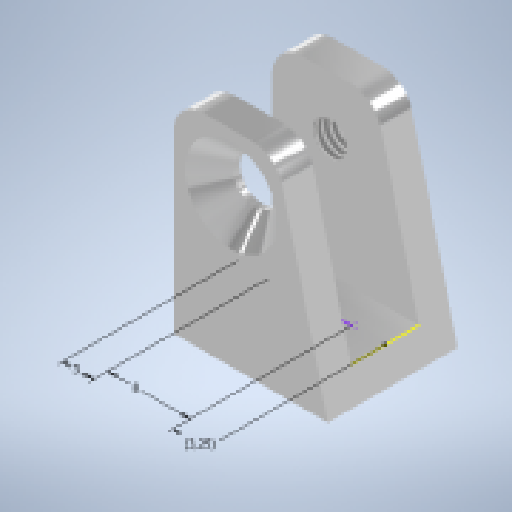
# Autodesk Inventor part: HalterUmlenkrolleH
Saved by Autodesk Inventor 2025 (Build 290162010, 162A)
## iProperties
Created: 2024-11-18
Part Number: HalterUmlenkrolleH
Material: Aluminium 6061(1)
Document SubType Name: Modeling
Designer: Admin
Density: 2.7 g/cm^3
Appearance: Aluminium - flach(1)
Author: Admin
Autodesk Inventor part; units mm, degrees
ref_plane "YZ Plane" through (0, 0, 0) normal (1, 0, 0) x (0, 1, 0)
ref_plane "XZ Plane" through (0, 0, 0) normal (0, 1, 0) x (-1, 0, 0)
ref_plane "XY Plane" through (0, 0, 0) normal (0, 0, 1) x (1, 0, 0)
sketch "Skizze1" plane through (0, 0, 0) normal (0, 0, 1) x (1, 0, 0)
  line L0 (17.8939, 18.6723) -> (2.8939, 18.6723)
  line L1 (2.8939, 18.6723) -> (2.8939, 15.6723)
  line L2 (2.8939, 15.6723) -> (17.8939, 15.6723)
  line L3 (17.8939, 15.6723) -> (17.8939, 18.6723)
  line L4 (17.8939, 9.0723) -> (2.8939, 9.0723)
  line L5 (2.8939, 9.0723) -> (2.8939, 6.0723)
  line L6 (2.8939, 6.0723) -> (17.8939, 6.0723)
  line L7 (17.8939, 6.0723) -> (17.8939, 9.0723)
  line L8 (17.8939, 15.6723) -> (17.8939, 12.3723) construction
  line L9 (17.8939, 12.3723) -> (17.8939, 9.0723) construction
  point P0 (0, 0)
  point P1 (10.3939, 9.0723)
  dimension "d0" = 15
  dimension "d1" = 3
  dimension "d2" = 3
  dimension "d3" = 6.6
  constraints: 20 end point, 5 equal length, 3 horizontal, 2 collinear, 2 perpendicular, 2 vertical, 1 midpoint
  measures "d0" distance of L2.end L1.end
  measures "d1" distance of L0.end L1.end
  measures "d2" distance of L4.end L5.end
  measures "d3" distance from line of point (10.394, 9.072) L2
extrude "Extrusion1" add sketch "Skizze1" along normal blind 20
chamfer "Fasen1" distance 5 distance2 20 1 edges at (17.8939, 7.5723, 20) measured on face at (17.3939, 7.5723, 20)
chamfer "Fasen2" distance 5 distance2 20 1 edges at (17.8939, 17.1723, 20) measured on face at (17.3939, 17.1723, 20)
fillet "Rundung1" radius 3 4 edges at (2.8939, 17.1723, 20) (2.8939, 7.5723, 20) (12.894, 17.1723, 20) (12.894, 7.5723, 20)
sketch "Skizze2" plane through (2.8939, 6.0723, 0) normal (0, -1, 0) x (1, 0, 0)
  circle A0 centre (5.6155, 14.3845) radius 5.6155 construction
  line L0 (0, 0) -> (0, 20) construction
  line L1 (5.6155, 14.3845) -> (5.6155, 20)
  line L2 (5.6155, 14.3845) -> (0, 14.3845)
  line L3 (3, 20) -> (7.6577, 20) projected
  line L4 (10.5681, 17.7276) -> (15, 0) projected
  point P0 (-2.8939, 0)
  point P1 (0, 17)
  constraints: 4 end point, 2 point on line, 2 vertical, 1 horizontal alignment, 1 perpendicular, 3 other
hole "Bohrung1" at (8.5094, 6.0723, 14.3845) direction (0, 1, 0) diameter 3.242 end through all countersink diameter 9 countersink angle 90 thread size "M4x0.7" class "6H" standard "ISO Metric profile"
sketch "Skizze3" plane through (2.8939, 15.6723, 0) normal (0, -1, 0) x (1, 0, 0)
  line L0 (0, 0) -> (15, 0) projected
  line L1 (15, 0) -> (14.25, 3)
  line L2 (14.25, 3) -> (0, 3)
  line L3 (0, 0) -> (0, 20) projected
  line L4 (15, 0) -> (10.5681, 17.7276) projected
  point P0 (-2.8939, 0)
  point P1 (0, 17)
  dimension "d51" = 3
  constraints: 4 end point, 2 point on line, 1 perpendicular
  measures "d51" distance between parallel lines of L0 L2
extrude "Extrusion2" add sketch "Skizze3" along normal through all
sketch "Skizze4" plane through (2.8939, 15.6723, 3) normal (0, 0, 1) x (1, 0, 0)
  line L0 (7.6577, 3) -> (3, 3) construction
  line L1 (3, -3.3) -> (11, -3.3)
  line L2 (3, -3.3) -> (0, -3.3)
  line L3 (14.25, 0) -> (14.25, -6.6) projected
  point P0 (12, 3)
  point P1 (14.25, -3.3)
  dimension "d48" = 8
  dimension "d49" = 3
  dimension "d50" = 3.25
  constraints: 4 end point, 2 horizontal, 1 coincident, 1 midpoint
  measures "d48" distance of L1.start L1.end
  measures "d49" distance of L1.start L2.end
  measures "d50" distance of point (14.25, -3.3) L1.end
sketch "Skizze5" plane through (2.8939, 6.0723, 0) normal (0, -1, 0) x (1, 0, 0)
  circle A0 centre (5.6155, 14.3845) radius 4.5 projected
  point P0 (-2.8939, 0)
  point P1 (11.255, 14.9799)
  point P2 (11.9803, 12.079)
  constraints: 1 other
hole "Bohrung3" at (8.5094, 6.0723, 14.3845) direction (0, 1, 0) diameter 4.3 depth 3 tip angle 118 clearance for "Flachkopfmaschinenschraube" size "M4" standard "ANSI Metrisches M Profil"
